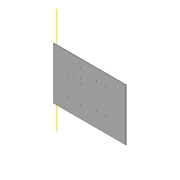
# Autodesk Inventor part: Board_Mounter
Saved by Autodesk Inventor 2020 (Build 240168000, 168)
## iProperties
Created: 2020-11-10
Part Number: Board_Mounter
Material: Generic
Document SubType Name: Modeling
Designer: magnarecta
Density: 1 g/cm^3
Appearance: Default
Author: magnarecta
Autodesk Inventor part; units mm, degrees
ref_plane "YZ Plane" through (0, 0, 0) normal (1, 0, 0) x (0, 1, 0)
ref_plane "XZ Plane" through (0, 0, 0) normal (0, 1, 0) x (-1, 0, 0)
ref_plane "XY Plane" through (0, 0, 0) normal (0, 0, 1) x (1, 0, 0)
ref_plane "Work Plane1" through (0, 0, 0) normal (0, 0, 1) x (1, 0, 0)
sketch "Sketch1" plane through (0, 0, 0) normal (0, 0, 1) x (1, 0, 0)
  line L0 (-18, 0) -> (-18, -560) projected
  line L1 (401, 0) -> (401, -560) projected
  line L2 (-19, 0) -> (-19, -560) projected
  circle A0 centre (64.8049, -277.2156) radius 1.8 projected
  circle A1 centre (64.8049, -379.0656) radius 1.8 projected
  circle A2 centre (140.9049, -379.0656) radius 1.8 projected
  circle A3 centre (140.9049, -277.2156) radius 1.8 projected
  circle A4 centre (138.1462, -248.6505) radius 1.5 projected
  circle A5 centre (138.1462, -196.6505) radius 1.5 projected
  circle A6 centre (96.1462, -248.6505) radius 1.5 projected
  circle A7 centre (96.1462, -196.6505) radius 1.5 projected
  circle A8 centre (231.6027, -214.3978) radius 2 projected
  circle A9 centre (281.6027, -214.3978) radius 2 projected
  circle A10 centre (281.6027, -364.3978) radius 2 projected
  circle A11 centre (231.6027, -364.3978) radius 2 projected
  line L3 (401, -150) -> (-19, -150)
  line L4 (-19, -150) -> (-19, -450)
  line L5 (-19, -450) -> (401, -450)
  line L6 (401, -450) -> (401, -150)
  point P0 (0, 0)
  point P1 (-18, -450)
  point P2 (-18, -150)
  dimension "d0" = 300
  dimension "d1" = 150
  constraints: 8 end point, 2 parallel, 2 point on line, 1 horizontal, 1 perpendicular
  measures "d0" distance between parallel lines of L5 L3
  measures "d1" distance from line of L3 L1.start
extrude "Extrusion1" add sketch "Sketch1" along normal blind 3 contours L3 L1 L5 L0
body "Solid1"
